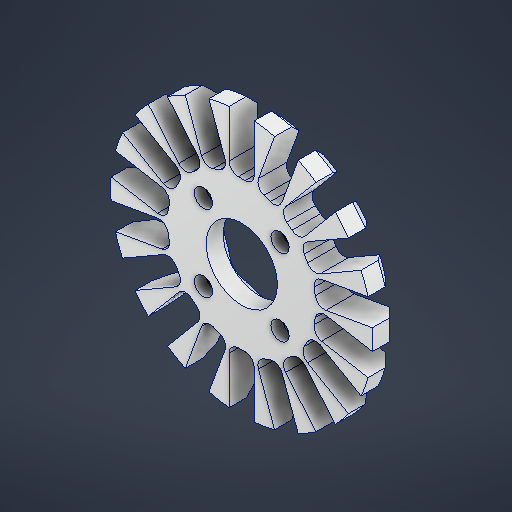
# Autodesk Inventor part: Raddeckel
Saved by Autodesk Inventor 2025.2 (Build 292293000, 293)
## iProperties
Created: 2025-03-24
Part Number: Raddeckel
Material: Generisch
Document SubType Name: Modeling
Designer: Faabs
Density: 1 g/cm^3
Appearance: Aluminium - flach
Author: Faabs
Autodesk Inventor part; units mm, degrees
ref_plane "YZ Plane" through (0, 0, 0) normal (1, 0, 0) x (0, 1, 0)
ref_plane "XZ Plane" through (0, 0, 0) normal (0, 1, 0) x (-1, 0, 0)
ref_plane "XY Plane" through (0, 0, 0) normal (0, 0, 1) x (1, 0, 0)
sketch "Skizze1" plane through (0, 0, 0) normal (0, 0, 1) x (1, 0, 0)
  line L0 (0, 0) -> (0, 5)
  line L1 (0, 0) -> (23, 0)
  line L2 (23, 0) -> (23, 3)
  line L3 (6.25, 0) -> (6.25, 5)
  line L4 (6.25, 5) -> (21, 5)
  line L5 (21, 5) -> (23, 3)
  dimension "d0" = 5
  dimension "d1" = 23
  dimension "d2" = 5
  dimension "d3" = 12.5
  dimension "d4" = 3
  dimension "d5" = 46
  dimension "d6" = 45
  constraints: 12 end point, 3 vertical, 2 horizontal, 2 point on line
  measures "d0" distance of L0.start L0.end
  measures "d1" distance of L0.start L1.end
  measures "d2" distance of L3.start L3.end
  measures "d3" diameter of L3 L0
  measures "d4" distance of L2.start L2.end
  measures "d5" diameter of L2 L0
  measures "d6" angle of L2 L5
revolve "Radkörper" add sketch "Skizze1" angle 360 about axis through (0, 0, 0) along (0, 1, 0)
sketch "Skizze2" plane through (0, 0, 0) normal (0, -1, 0) x (1, 0, 0)
  circle A0 centre (0, 0) radius 23
  circle A1 centre (0, 0) radius 13 construction
  line L0 (0, 0) -> (0, 23) construction
  line L1 (0, 23) -> (2.2, 23)
  line L2 (2.2, 23) -> (2.2, 14.6)
  line L3 (0.6, 13) -> (0, 13)
  line L4 (0, 13) -> (0, 23) construction
  line L5 (0, 23) -> (-2.2, 23)
  line L6 (-2.2, 23) -> (-2.2, 14.6)
  line L7 (-0.6, 13) -> (0, 13)
  line L8 (0, 13) -> (0, 23) construction
  arc A2 (-2.2, 14.6) -> (-0.6, 13) centre (-0.6, 14.6) ccw
  arc A3 (0.6, 13) -> (2.2, 14.6) centre (0.6, 14.6) ccw
  point P0 (2.2, 13)
  point P1 (-2.2, 13)
  point P2 (2.2, 22.8945)
  point P3 (-2.2, 22.8945)
  point P4 (0, 13)
  dimension "d8" = 46
  dimension "d9" = 26
  dimension "d10" = 2.2
  dimension "d12" = 4.4
  dimension "d15" = 1.6
  dimension "d46" = 8.4
  dimension "d47" = 8.4
  constraints: 18 end point, 4 parallel, 4 point on circle, 4 point on line, 4 tangent, 3 centre point, 2 coincident, 2 horizontal, 2 perpendicular, 1 equal radius, 1 vertical, 3 other
  measures "d9" diameter of A1
  measures "d10" distance of point (2.2, 13) L3.end
  measures "d12" distance between parallel lines of L6 L2
  measures "d15" radius of A2
  measures "d46" distance from line of L1 A3.centre
  measures "d47" distance from line of A2.centre L5
extrude "Querrolle" cut sketch "Skizze2" against normal up to surface (5 mm away) contours L2 A3 L3 L7 A2 L6 A0 picked at (0, 17.4)
pattern_circular "Runde Anordnung1" count 18 over 360 about axis through (0, -10, 0) along (0, 1, 0) of "Querrolle"
sketch "Skizze3" plane through (-2.2, 5, 20.8844) normal (0, 1, 0) x (1, 0, 0)
  circle A0 centre (2.2, 20.8844) radius 9.5 construction
  line L0 (2.2, 20.8844) -> (2.2, 11.3844) construction
  line L1 (2.2, 20.8844) -> (8.9175, 14.1669) construction
  point P0 (8.9175, 27.602)
  point P1 (-4.5175, 27.602)
  point P2 (-4.5175, 14.1669)
  dimension "d21" = 19
  dimension "d22" = 45
  dimension "d25" = 360
  constraints: 4 end point, 2 coincident, 2 point on circle, 1 centre point, 1 vertical, 5 other
  measures "d21" diameter of A0
  measures "d22" angle of L1 L0
hole "Bohrung1" at (6.7175, 5, 6.7175) at (6.7175, 5, -6.7175) at (-6.7175, 5, -6.7175) at (-6.7175, 5, 6.7175) direction (0, -1, 0) diameter 3.2 depth 5 tip angle 118 counterbore diameter 5.6 counterbore depth 3
chamfer "Fasen5" distance 2 angle 45 1 edges at (-6.25, 5, 0)
chamfer "Fasen6" distance 0.25 angle 45 6 edges at (-4.9297, 5, 8.8724) (-9.5055, 5, 6.9771) (4.9297, 5, 8.8724) (9.5055, 5, 6.9771) (-8.6974, 5, -8.6974) (8.6974, 5, -8.6974)
sketch "Skizze5" plane through (-2.2, 5, 20.8844) normal (0, 1, 0) x (1, 0, 0)
  circle A0 centre (2.2, 20.8844) radius 6.25
  constraints: 1 centre point, 1 coincident
extrude "Extrusion3" [suppressed]
sketch "Skizze6" plane through (-2.2, 5, 20.8844) normal (0, 1, 0) x (1, 0, 0)
  circle A0 centre (3.6842, 23.4177) radius 1
  circle A1 centre (4.7424, 19.8077) radius 1
  circle A2 centre (1.6362, 17.6858) radius 1
  circle A3 centre (-1.3418, 19.9843) radius 1
  circle A4 centre (-0.076, 23.5268) radius 1
  circle A5 centre (1.729, 20.8844) radius 1.6
  line L0 (1.729, 20.8844) -> (2.2, 20.8844)
  circle A6 centre (1.729, 20.8844) radius 1.6
  spline S0 degree 5 poles (4.0455, 16.9262) (4.0402, 16.9231) (4.0297, 16.9169) (4.014, 16.9073) (3.9934, 16.894) (3.9682, 16.8764) (3.9436, 16.8581) (3.9196, 16.8389) (3.8963, 16.8192) (3.8739, 16.799) (3.8525, 16.7785) (3.8322, 16.758) (3.813, 16.7376) (3.7948, 16.7171) (3.7774, 16.6963) (3.7607, 16.675) (3.7442, 16.6528) (3.7279, 16.6295) (3.7116, 16.6049) (3.6956, 16.579) (3.6799, 16.5519) (3.6648, 16.5239) (3.6505, 16.4953) (3.6371, 16.4663) (3.6248, 16.4374) (3.6136, 16.4089) (3.6035, 16.3809) (3.5944, 16.3536) (3.5861, 16.3267) (3.5786, 16.2999) (3.5716, 16.2728) (3.565, 16.2453) (3.5586, 16.2172) (3.5524, 16.1887) (3.5463, 16.1602) (3.5403, 16.132) (3.534, 16.1044) (3.527, 16.0771) (3.5186, 16.0497) (3.5081, 16.0214) (3.495, 15.9919) (3.4788, 15.9607) (3.4596, 15.928) (3.4382, 15.8946) (3.4152, 15.8615) (3.3915, 15.8297) (3.368, 15.8004) (3.3452, 15.774) (3.3233, 15.7507) (3.302, 15.73) (3.2808, 15.7111) (3.2589, 15.693) (3.2359, 15.675) (3.2114, 15.6567) (3.1855, 15.6381) (3.1584, 15.6194) (3.1303, 15.601) (3.1015, 15.5835) (3.0723, 15.5669) (3.0427, 15.5515) (3.0127, 15.5372) (2.9823, 15.5238) (2.9513, 15.5112) (2.9198, 15.4994) (2.8876, 15.4883) (2.855, 15.4779) (2.822, 15.4683) (2.7887, 15.4596) (2.7552, 15.4518) (2.7215, 15.445) (2.6876, 15.4393) (2.6536, 15.4346) (2.6196, 15.4309) (2.5854, 15.4283) (2.5512, 15.4266) (2.517, 15.4258) (2.483, 15.426) (2.4493, 15.427) (2.4158, 15.4288) (2.3827, 15.4316) (2.3499, 15.4352) (2.3173, 15.4399) (2.285, 15.4457) (2.2528, 15.4525) (2.221, 15.4604) (2.1895, 15.4692) (2.1589, 15.4787) (2.1292, 15.4885) (2.1009, 15.4987) (2.0737, 15.5091) (2.0476, 15.52) (2.022, 15.5318) (1.9962, 15.545) (1.9698, 15.56) (1.9426, 15.5769) (1.9149, 15.5955) (1.8875, 15.6151) (1.8612, 15.635) (1.8369, 15.6545) (1.815, 15.6734) (1.7956, 15.6918) (1.778, 15.7104) (1.7615, 15.7301) (1.7452, 15.7516) (1.7285, 15.7754) (1.7111, 15.8014) (1.693, 15.829) (1.6745, 15.8575) (1.6557, 15.8862) (1.6368, 15.9144) (1.6177, 15.9418) (1.598, 15.9686) (1.5775, 15.9948) (1.5559, 16.0206) (1.5331, 16.0461) (1.5093, 16.0711) (1.4849, 16.0953) (1.4605, 16.1182) (1.4366, 16.1394) (1.4135, 16.1587) (1.3913, 16.1761) (1.3698, 16.1919) (1.3485, 16.2067) (1.3267, 16.2209) (1.3039, 16.2351) (1.2796, 16.2494) (1.2537, 16.2637) (1.2259, 16.2778) (1.1964, 16.2915) (1.1657, 16.3044) (1.1343, 16.3164) (1.1031, 16.3272) (1.0728, 16.3367) (1.0443, 16.3449) (1.0183, 16.3517) (0.9953, 16.3571) (0.9793, 16.3603) (0.9687, 16.362) (0.9623, 16.3629) (0.9593, 16.3632) knots 0 0 0 0 0 0 0.007407 0.014815 0.022222 0.02963 0.037037 0.044444 0.051852 0.059259 0.066667 0.074074 0.081481 0.088889 0.096296 0.103704 0.111111 0.118519 0.125926 0.133333 0.140741 0.148148 0.155556 0.162963 0.17037 0.177778 0.185185 0.192593 0.2 0.207407 0.214815 0.222222 0.22963 0.237037 0.244444 0.251852 0.259259 0.266667 0.274074 0.281481 0.288889 0.296296 0.303704 0.311111 0.318519 0.325926 0.333333 0.340741 0.348148 0.355556 0.362963 0.37037 0.377778 0.385185 0.392593 0.4 0.407407 0.414815 0.422222 0.42963 0.437037 0.444444 0.451852 0.459259 0.466667 0.474074 0.481481 0.488889 0.496296 0.503704 0.511111 0.518519 0.525926 0.533333 0.540741 0.548148 0.555556 0.562963 0.57037 0.577778 0.585185 0.592593 0.6 0.607407 0.614815 0.622222 0.62963 0.637037 0.644444 0.651852 0.659259 0.666667 0.674074 0.681481 0.688889 0.696296 0.703704 0.711111 0.718519 0.725926 0.733333 0.740741 0.748148 0.755556 0.762963 0.77037 0.777778 0.785185 0.792593 0.8 0.807407 0.814815 0.822222 0.82963 0.837037 0.844444 0.851852 0.859259 0.866667 0.874074 0.881481 0.888889 0.896296 0.903704 0.911111 0.918519 0.925926 0.933333 0.940741 0.948148 0.955556 0.962963 0.97037 0.977778 0.985185 0.992593 1 1 1 1 1 1
  spline S1 degree 5 poles (0.9593, 16.3632) (0.9532, 16.3643) (0.9411, 16.3663) (0.9229, 16.369) (0.8986, 16.3721) (0.868, 16.3748) (0.8374, 16.3766) (0.8067, 16.3773) (0.7762, 16.3771) (0.746, 16.3761) (0.7165, 16.3742) (0.6877, 16.3715) (0.6598, 16.3682) (0.6327, 16.3642) (0.6061, 16.3594) (0.5796, 16.3539) (0.5527, 16.3475) (0.5252, 16.3401) (0.4969, 16.3317) (0.468, 16.3222) (0.4386, 16.3116) (0.409, 16.2998) (0.3796, 16.2871) (0.3508, 16.2735) (0.3228, 16.2592) (0.2959, 16.2445) (0.2701, 16.2296) (0.2456, 16.2145) (0.222, 16.1992) (0.199, 16.1836) (0.1762, 16.1674) (0.1534, 16.1505) (0.1305, 16.1331) (0.1074, 16.1152) (0.0845, 16.0973) (0.0617, 16.0796) (0.0391, 16.0624) (0.0162, 16.046) (-0.0078, 16.0304) (-0.034, 16.0156) (-0.0631, 16.0014) (-0.0956, 15.9879) (-0.1312, 15.9751) (-0.1691, 15.9633) (-0.208, 15.9528) (-0.2466, 15.9437) (-0.2835, 15.9363) (-0.3178, 15.9307) (-0.3496, 15.927) (-0.3792, 15.9248) (-0.4076, 15.924) (-0.436, 15.9242) (-0.4652, 15.9252) (-0.4957, 15.9269) (-0.5276, 15.9293) (-0.5604, 15.9324) (-0.5937, 15.9364) (-0.627, 15.9414) (-0.66, 15.9475) (-0.6926, 15.9547) (-0.7248, 15.963) (-0.7567, 15.9723) (-0.7885, 15.9826) (-0.8203, 15.9939) (-0.852, 16.006) (-0.8837, 16.019) (-0.9151, 16.0328) (-0.9463, 16.0476) (-0.977, 16.0632) (-1.0071, 16.0797) (-1.0367, 16.097) (-1.0658, 16.1153) (-1.0942, 16.1344) (-1.1221, 16.1543) (-1.1494, 16.175) (-1.1761, 16.1964) (-1.202, 16.2183) (-1.2273, 16.2408) (-1.2517, 16.2637) (-1.2753, 16.2871) (-1.2981, 16.311) (-1.32, 16.3355) (-1.3411, 16.3607) (-1.3613, 16.3866) (-1.3806, 16.4132) (-1.3991, 16.4401) (-1.4165, 16.4671) (-1.4328, 16.4937) (-1.448, 16.5197) (-1.4621, 16.5451) (-1.4751, 16.5702) (-1.4872, 16.5957) (-1.4985, 16.6224) (-1.5091, 16.6509) (-1.519, 16.6814) (-1.5283, 16.7134) (-1.5367, 16.746) (-1.544, 16.7781) (-1.5501, 16.8088) (-1.5547, 16.8373) (-1.5578, 16.8639) (-1.5592, 16.8894) (-1.5592, 16.9151) (-1.5579, 16.942) (-1.5554, 16.971) (-1.552, 17.0021) (-1.5481, 17.0349) (-1.544, 17.0686) (-1.54, 17.1026) (-1.5363, 17.1364) (-1.5333, 17.1697) (-1.5312, 17.2029) (-1.5301, 17.2361) (-1.53, 17.2698) (-1.5311, 17.304) (-1.5333, 17.3384) (-1.5364, 17.3726) (-1.5404, 17.4058) (-1.545, 17.4375) (-1.5503, 17.4671) (-1.5561, 17.4947) (-1.5624, 17.5206) (-1.5693, 17.5457) (-1.5768, 17.5706) (-1.5852, 17.5961) (-1.5946, 17.6226) (-1.6053, 17.6503) (-1.6175, 17.679) (-1.6313, 17.7084) (-1.6465, 17.738) (-1.6628, 17.7674) (-1.6798, 17.7957) (-1.6969, 17.8225) (-1.7134, 17.8471) (-1.729, 17.869) (-1.7432, 17.888) (-1.7534, 17.9006) (-1.7604, 17.9088) (-1.7647, 17.9135) (-1.7668, 17.9158) knots 0 0 0 0 0 0 0.007407 0.014815 0.022222 0.02963 0.037037 0.044444 0.051852 0.059259 0.066667 0.074074 0.081481 0.088889 0.096296 0.103704 0.111111 0.118519 0.125926 0.133333 0.140741 0.148148 0.155556 0.162963 0.17037 0.177778 0.185185 0.192593 0.2 0.207407 0.214815 0.222222 0.22963 0.237037 0.244444 0.251852 0.259259 0.266667 0.274074 0.281481 0.288889 0.296296 0.303704 0.311111 0.318519 0.325926 0.333333 0.340741 0.348148 0.355556 0.362963 0.37037 0.377778 0.385185 0.392593 0.4 0.407407 0.414815 0.422222 0.42963 0.437037 0.444444 0.451852 0.459259 0.466667 0.474074 0.481481 0.488889 0.496296 0.503704 0.511111 0.518519 0.525926 0.533333 0.540741 0.548148 0.555556 0.562963 0.57037 0.577778 0.585185 0.592593 0.6 0.607407 0.614815 0.622222 0.62963 0.637037 0.644444 0.651852 0.659259 0.666667 0.674074 0.681481 0.688889 0.696296 0.703704 0.711111 0.718519 0.725926 0.733333 0.740741 0.748148 0.755556 0.762963 0.77037 0.777778 0.785185 0.792593 0.8 0.807407 0.814815 0.822222 0.82963 0.837037 0.844444 0.851852 0.859259 0.866667 0.874074 0.881481 0.888889 0.896296 0.903704 0.911111 0.918519 0.925926 0.933333 0.940741 0.948148 0.955556 0.962963 0.97037 0.977778 0.985185 0.992593 1 1 1 1 1 1
  spline S2 degree 5 poles (-1.7668, 17.9158) (-1.7708, 17.9205) (-1.7787, 17.9298) (-1.7909, 17.9436) (-1.8076, 17.9615) (-1.8293, 17.9833) (-1.8516, 18.0043) (-1.8747, 18.0246) (-1.8982, 18.0441) (-1.9219, 18.0627) (-1.9458, 18.0802) (-1.9695, 18.0967) (-1.993, 18.112) (-2.0164, 18.1264) (-2.0398, 18.1399) (-2.0637, 18.1527) (-2.0884, 18.165) (-2.1142, 18.1771) (-2.1413, 18.1888) (-2.1696, 18.2001) (-2.1989, 18.2109) (-2.2291, 18.2209) (-2.2598, 18.23) (-2.2906, 18.2381) (-2.3213, 18.2452) (-2.3513, 18.2513) (-2.3806, 18.2564) (-2.4091, 18.2606) (-2.4371, 18.2641) (-2.4647, 18.2668) (-2.4926, 18.269) (-2.5208, 18.2708) (-2.5497, 18.2722) (-2.5788, 18.2734) (-2.6079, 18.2744) (-2.6367, 18.2754) (-2.665, 18.2768) (-2.6931, 18.2789) (-2.7216, 18.2825) (-2.7512, 18.2879) (-2.7826, 18.2957) (-2.8161, 18.3063) (-2.8516, 18.3194) (-2.8883, 18.3347) (-2.9249, 18.3517) (-2.9602, 18.3695) (-2.9932, 18.3875) (-3.0232, 18.4054) (-3.0499, 18.4229) (-3.0739, 18.4402) (-3.0963, 18.4579) (-3.1179, 18.4763) (-3.1396, 18.4958) (-3.1619, 18.5168) (-3.1848, 18.539) (-3.2079, 18.5625) (-3.2308, 18.587) (-3.2531, 18.6123) (-3.2745, 18.6381) (-3.2948, 18.6646) (-3.3141, 18.6917) (-3.3326, 18.7193) (-3.3503, 18.7476) (-3.3675, 18.7767) (-3.384, 18.8064) (-3.3999, 18.8367) (-3.4151, 18.8675) (-3.4295, 18.8988) (-3.4429, 18.9305) (-3.4555, 18.9625) (-3.467, 18.9949) (-3.4775, 19.0275) (-3.487, 19.0604) (-3.4956, 19.0936) (-3.5032, 19.127) (-3.5099, 19.1605) (-3.5156, 19.194) (-3.5205, 19.2274) (-3.5245, 19.2607) (-3.5275, 19.2938) (-3.5296, 19.3267) (-3.5307, 19.3596) (-3.5306, 19.3925) (-3.5294, 19.4253) (-3.5272, 19.4581) (-3.524, 19.4906) (-3.52, 19.5224) (-3.5154, 19.5533) (-3.5104, 19.583) (-3.5049, 19.6115) (-3.4987, 19.6391) (-3.4915, 19.6664) (-3.483, 19.6941) (-3.4728, 19.7228) (-3.4608, 19.7525) (-3.4473, 19.783) (-3.4328, 19.8134) (-3.4178, 19.8427) (-3.4027, 19.8701) (-3.3879, 19.8949) (-3.3732, 19.9172) (-3.3579, 19.9377) (-3.3414, 19.9574) (-3.323, 19.9771) (-3.3025, 19.9977) (-3.2799, 20.0194) (-3.2559, 20.042) (-3.231, 20.0652) (-3.2061, 20.0886) (-3.1816, 20.1122) (-3.1579, 20.1358) (-3.1349, 20.1598) (-3.1127, 20.1846) (-3.091, 20.2103) (-3.0699, 20.2372) (-3.0494, 20.265) (-3.0298, 20.2932) (-3.0115, 20.3212) (-2.9947, 20.3484) (-2.9797, 20.3745) (-2.9665, 20.3994) (-2.9546, 20.4233) (-2.9438, 20.4469) (-2.9335, 20.4708) (-2.9235, 20.4957) (-2.9137, 20.5221) (-2.9041, 20.5502) (-2.895, 20.58) (-2.8866, 20.6114) (-2.8792, 20.6439) (-2.8729, 20.6769) (-2.8677, 20.7095) (-2.8636, 20.741) (-2.8604, 20.7704) (-2.8583, 20.7972) (-2.857, 20.8209) (-2.8566, 20.8372) (-2.8568, 20.8479) (-2.857, 20.8543) (-2.8572, 20.8574) knots 0 0 0 0 0 0 0.007407 0.014815 0.022222 0.02963 0.037037 0.044444 0.051852 0.059259 0.066667 0.074074 0.081481 0.088889 0.096296 0.103704 0.111111 0.118519 0.125926 0.133333 0.140741 0.148148 0.155556 0.162963 0.17037 0.177778 0.185185 0.192593 0.2 0.207407 0.214815 0.222222 0.22963 0.237037 0.244444 0.251852 0.259259 0.266667 0.274074 0.281481 0.288889 0.296296 0.303704 0.311111 0.318519 0.325926 0.333333 0.340741 0.348148 0.355556 0.362963 0.37037 0.377778 0.385185 0.392593 0.4 0.407407 0.414815 0.422222 0.42963 0.437037 0.444444 0.451852 0.459259 0.466667 0.474074 0.481481 0.488889 0.496296 0.503704 0.511111 0.518519 0.525926 0.533333 0.540741 0.548148 0.555556 0.562963 0.57037 0.577778 0.585185 0.592593 0.6 0.607407 0.614815 0.622222 0.62963 0.637037 0.644444 0.651852 0.659259 0.666667 0.674074 0.681481 0.688889 0.696296 0.703704 0.711111 0.718519 0.725926 0.733333 0.740741 0.748148 0.755556 0.762963 0.77037 0.777778 0.785185 0.792593 0.8 0.807407 0.814815 0.822222 0.82963 0.837037 0.844444 0.851852 0.859259 0.866667 0.874074 0.881481 0.888889 0.896296 0.903704 0.911111 0.918519 0.925926 0.933333 0.940741 0.948148 0.955556 0.962963 0.97037 0.977778 0.985185 0.992593 1 1 1 1 1 1
  spline S3 degree 5 poles (-2.8572, 20.8574) (-2.8572, 20.8635) (-2.8573, 20.8758) (-2.8578, 20.8942) (-2.859, 20.9187) (-2.8616, 20.9493) (-2.8652, 20.9798) (-2.8698, 21.0101) (-2.8753, 21.0401) (-2.8816, 21.0696) (-2.8886, 21.0984) (-2.8962, 21.1262) (-2.9043, 21.1531) (-2.913, 21.1791) (-2.9223, 21.2045) (-2.9323, 21.2297) (-2.9433, 21.2551) (-2.9553, 21.2809) (-2.9685, 21.3072) (-2.9829, 21.3341) (-2.9985, 21.3612) (-3.0152, 21.3883) (-3.0328, 21.415) (-3.0512, 21.441) (-3.0701, 21.4661) (-3.0893, 21.4901) (-3.1084, 21.5128) (-3.1276, 21.5344) (-3.1467, 21.555) (-3.1662, 21.5749) (-3.1861, 21.5945) (-3.2066, 21.614) (-3.2278, 21.6336) (-3.2493, 21.6532) (-3.271, 21.6727) (-3.2924, 21.692) (-3.3132, 21.7113) (-3.3333, 21.731) (-3.3529, 21.752) (-3.372, 21.7752) (-3.3911, 21.8014) (-3.41, 21.831) (-3.4287, 21.8639) (-3.4469, 21.8992) (-3.4641, 21.9357) (-3.4798, 21.972) (-3.4934, 22.0071) (-3.5049, 22.04) (-3.5141, 22.0706) (-3.5214, 22.0994) (-3.5271, 22.1272) (-3.5319, 22.1552) (-3.5359, 22.1841) (-3.5396, 22.2145) (-3.5428, 22.2463) (-3.5454, 22.2791) (-3.5472, 22.3126) (-3.548, 22.3463) (-3.5478, 22.3798) (-3.5463, 22.4132) (-3.5438, 22.4463) (-3.5401, 22.4794) (-3.5355, 22.5125) (-3.53, 22.5457) (-3.5235, 22.5791) (-3.5162, 22.6126) (-3.5081, 22.6459) (-3.4989, 22.6792) (-3.4889, 22.7121) (-3.4779, 22.7447) (-3.466, 22.7768) (-3.453, 22.8086) (-3.4392, 22.84) (-3.4244, 22.8709) (-3.4087, 22.9013) (-3.3923, 22.9313) (-3.3752, 22.9607) (-3.3575, 22.9894) (-3.3391, 23.0175) (-3.3202, 23.0448) (-3.3006, 23.0714) (-3.2803, 23.0972) (-3.2591, 23.1223) (-3.2371, 23.1467) (-3.2143, 23.1704) (-3.191, 23.1932) (-3.1675, 23.2151) (-3.1441, 23.2358) (-3.1211, 23.2553) (-3.0986, 23.2736) (-3.0761, 23.2907) (-3.053, 23.3071) (-3.0287, 23.3228) (-3.0025, 23.3382) (-2.9742, 23.3533) (-2.9443, 23.3679) (-2.9136, 23.3819) (-2.8833, 23.3947) (-2.8542, 23.406) (-2.8269, 23.4155) (-2.8012, 23.4231) (-2.7763, 23.429) (-2.7511, 23.4334) (-2.7243, 23.4368) (-2.6953, 23.4394) (-2.6641, 23.4415) (-2.6311, 23.4433) (-2.5972, 23.4451) (-2.563, 23.447) (-2.5291, 23.4493) (-2.4958, 23.4522) (-2.4628, 23.4558) (-2.4298, 23.4605) (-2.3967, 23.4663) (-2.3632, 23.4733) (-2.3297, 23.4814) (-2.2965, 23.4904) (-2.2645, 23.5001) (-2.2341, 23.5102) (-2.2059, 23.5205) (-2.1797, 23.531) (-2.1553, 23.5418) (-2.1318, 23.5529) (-2.1086, 23.5646) (-2.0849, 23.5773) (-2.0604, 23.5911) (-2.035, 23.6065) (-2.0089, 23.6235) (-1.9823, 23.6421) (-1.9557, 23.6623) (-1.9297, 23.6835) (-1.9047, 23.7052) (-1.8813, 23.7266) (-1.86, 23.7471) (-1.8411, 23.7662) (-1.8249, 23.7835) (-1.8142, 23.7958) (-1.8074, 23.8041) (-1.8035, 23.8092) (-1.8016, 23.8117) knots 0 0 0 0 0 0 0.007407 0.014815 0.022222 0.02963 0.037037 0.044444 0.051852 0.059259 0.066667 0.074074 0.081481 0.088889 0.096296 0.103704 0.111111 0.118519 0.125926 0.133333 0.140741 0.148148 0.155556 0.162963 0.17037 0.177778 0.185185 0.192593 0.2 0.207407 0.214815 0.222222 0.22963 0.237037 0.244444 0.251852 0.259259 0.266667 0.274074 0.281481 0.288889 0.296296 0.303704 0.311111 0.318519 0.325926 0.333333 0.340741 0.348148 0.355556 0.362963 0.37037 0.377778 0.385185 0.392593 0.4 0.407407 0.414815 0.422222 0.42963 0.437037 0.444444 0.451852 0.459259 0.466667 0.474074 0.481481 0.488889 0.496296 0.503704 0.511111 0.518519 0.525926 0.533333 0.540741 0.548148 0.555556 0.562963 0.57037 0.577778 0.585185 0.592593 0.6 0.607407 0.614815 0.622222 0.62963 0.637037 0.644444 0.651852 0.659259 0.666667 0.674074 0.681481 0.688889 0.696296 0.703704 0.711111 0.718519 0.725926 0.733333 0.740741 0.748148 0.755556 0.762963 0.77037 0.777778 0.785185 0.792593 0.8 0.807407 0.814815 0.822222 0.82963 0.837037 0.844444 0.851852 0.859259 0.866667 0.874074 0.881481 0.888889 0.896296 0.903704 0.911111 0.918519 0.925926 0.933333 0.940741 0.948148 0.955556 0.962963 0.97037 0.977778 0.985185 0.992593 1 1 1 1 1 1
  spline S4 degree 5 poles (-1.8016, 23.8117) (-1.7977, 23.8164) (-1.7899, 23.8258) (-1.7784, 23.8402) (-1.7636, 23.8598) (-1.746, 23.8849) (-1.7291, 23.9106) (-1.7131, 23.9367) (-1.698, 23.9633) (-1.6839, 23.9899) (-1.6708, 24.0164) (-1.6587, 24.0427) (-1.6476, 24.0685) (-1.6375, 24.094) (-1.6283, 24.1194) (-1.6199, 24.1452) (-1.612, 24.1717) (-1.6046, 24.1992) (-1.5978, 24.2278) (-1.5915, 24.2577) (-1.586, 24.2884) (-1.5814, 24.3199) (-1.5778, 24.3517) (-1.5751, 24.3835) (-1.5735, 24.4149) (-1.5727, 24.4455) (-1.5728, 24.4753) (-1.5736, 24.5041) (-1.575, 24.5322) (-1.5771, 24.5599) (-1.5797, 24.5877) (-1.5829, 24.6159) (-1.5865, 24.6445) (-1.5905, 24.6734) (-1.5945, 24.7022) (-1.5985, 24.7308) (-1.6021, 24.7589) (-1.6048, 24.7869) (-1.6063, 24.8156) (-1.6061, 24.8457) (-1.6038, 24.878) (-1.5993, 24.9128) (-1.5925, 24.9501) (-1.5837, 24.9888) (-1.5734, 25.0278) (-1.5621, 25.0657) (-1.55, 25.1014) (-1.5376, 25.1339) (-1.525, 25.1633) (-1.5121, 25.19) (-1.4986, 25.2151) (-1.4842, 25.2395) (-1.4687, 25.2643) (-1.452, 25.2899) (-1.4341, 25.3163) (-1.4149, 25.3431) (-1.3948, 25.37) (-1.3738, 25.3963) (-1.352, 25.4218) (-1.3295, 25.4464) (-1.3062, 25.4702) (-1.2822, 25.4932) (-1.2574, 25.5156) (-1.2318, 25.5375) (-1.2054, 25.5589) (-1.1783, 25.5798) (-1.1506, 25.6001) (-1.1222, 25.6197) (-1.0934, 25.6385) (-1.064, 25.6564) (-1.0342, 25.6734) (-1.0038, 25.6894) (-0.9731, 25.7045) (-0.9419, 25.7187) (-0.9103, 25.732) (-0.8785, 25.7444) (-0.8465, 25.7559) (-0.8144, 25.7665) (-0.7823, 25.7762) (-0.7503, 25.7849) (-0.7182, 25.7927) (-0.686, 25.7994) (-0.6536, 25.8051) (-0.6211, 25.8096) (-0.5884, 25.8131) (-0.5559, 25.8156) (-0.5238, 25.8172) (-0.4926, 25.8181) (-0.4625, 25.8182) (-0.4335, 25.8177) (-0.4052, 25.8165) (-0.377, 25.8141) (-0.3483, 25.8105) (-0.3183, 25.8055) (-0.287, 25.7988) (-0.2546, 25.7909) (-0.2222, 25.7818) (-0.1907, 25.7721) (-0.1611, 25.7621) (-0.1341, 25.7518) (-0.1095, 25.7412) (-0.0867, 25.7297) (-0.0645, 25.7168) (-0.0418, 25.7022) (-0.0179, 25.6855) (0.0073, 25.6671) (0.0337, 25.6473) (0.0609, 25.6269) (0.0883, 25.6064) (0.1157, 25.5863) (0.1431, 25.5671) (0.1708, 25.5487) (0.199, 25.5311) (0.2281, 25.5142) (0.2582, 25.498) (0.2892, 25.4827) (0.3203, 25.4683) (0.3511, 25.4551) (0.3809, 25.4433) (0.4092, 25.4331) (0.4359, 25.4243) (0.4616, 25.4168) (0.4867, 25.4103) (0.512, 25.4043) (0.5383, 25.3988) (0.566, 25.3937) (0.5953, 25.3891) (0.6262, 25.3854) (0.6586, 25.3826) (0.6919, 25.3809) (0.7255, 25.3804) (0.7585, 25.381) (0.7902, 25.3823) (0.8198, 25.3844) (0.8465, 25.3869) (0.87, 25.3897) (0.8861, 25.3922) (0.8967, 25.3942) (0.903, 25.3956) (0.906, 25.3963) knots 0 0 0 0 0 0 0.007407 0.014815 0.022222 0.02963 0.037037 0.044444 0.051852 0.059259 0.066667 0.074074 0.081481 0.088889 0.096296 0.103704 0.111111 0.118519 0.125926 0.133333 0.140741 0.148148 0.155556 0.162963 0.17037 0.177778 0.185185 0.192593 0.2 0.207407 0.214815 0.222222 0.22963 0.237037 0.244444 0.251852 0.259259 0.266667 0.274074 0.281481 0.288889 0.296296 0.303704 0.311111 0.318519 0.325926 0.333333 0.340741 0.348148 0.355556 0.362963 0.37037 0.377778 0.385185 0.392593 0.4 0.407407 0.414815 0.422222 0.42963 0.437037 0.444444 0.451852 0.459259 0.466667 0.474074 0.481481 0.488889 0.496296 0.503704 0.511111 0.518519 0.525926 0.533333 0.540741 0.548148 0.555556 0.562963 0.57037 0.577778 0.585185 0.592593 0.6 0.607407 0.614815 0.622222 0.62963 0.637037 0.644444 0.651852 0.659259 0.666667 0.674074 0.681481 0.688889 0.696296 0.703704 0.711111 0.718519 0.725926 0.733333 0.740741 0.748148 0.755556 0.762963 0.77037 0.777778 0.785185 0.792593 0.8 0.807407 0.814815 0.822222 0.82963 0.837037 0.844444 0.851852 0.859259 0.866667 0.874074 0.881481 0.888889 0.896296 0.903704 0.911111 0.918519 0.925926 0.933333 0.940741 0.948148 0.955556 0.962963 0.97037 0.977778 0.985185 0.992593 1 1 1 1 1 1
  spline S5 degree 5 poles (0.906, 25.3963) (0.912, 25.3973) (0.9241, 25.3996) (0.9421, 25.4032) (0.966, 25.4087) (0.9957, 25.4166) (1.0251, 25.4254) (1.0542, 25.4352) (1.0828, 25.4458) (1.1107, 25.4571) (1.1379, 25.469) (1.164, 25.4813) (1.189, 25.494) (1.2131, 25.507) (1.2365, 25.5206) (1.2596, 25.5349) (1.2826, 25.5501) (1.306, 25.5665) (1.3297, 25.584) (1.3536, 25.6029) (1.3776, 25.6229) (1.4014, 25.644) (1.4246, 25.6661) (1.447, 25.6887) (1.4685, 25.7117) (1.4888, 25.7347) (1.5078, 25.7575) (1.5258, 25.7801) (1.5427, 25.8026) (1.559, 25.8251) (1.5748, 25.8481) (1.5904, 25.8717) (1.6061, 25.896) (1.6216, 25.9206) (1.6371, 25.9454) (1.6524, 25.9698) (1.6677, 25.9936) (1.6836, 26.0169) (1.7009, 26.0397) (1.7204, 26.0627) (1.7429, 26.0859) (1.7688, 26.1097) (1.7979, 26.1339) (1.8295, 26.158) (1.8625, 26.1812) (1.8956, 26.2029) (1.9277, 26.2225) (1.9581, 26.2395) (1.9867, 26.2539) (2.0137, 26.266) (2.0402, 26.2765) (2.0669, 26.286) (2.0947, 26.2951) (2.124, 26.3039) (2.1547, 26.3126) (2.1866, 26.3209) (2.2193, 26.3285) (2.2523, 26.3352) (2.2854, 26.3407) (2.3185, 26.3451) (2.3516, 26.3483) (2.3847, 26.3505) (2.4182, 26.3517) (2.4519, 26.352) (2.4858, 26.3515) (2.52, 26.3501) (2.5543, 26.3478) (2.5886, 26.3446) (2.6228, 26.3404) (2.6568, 26.3353) (2.6906, 26.3291) (2.7241, 26.3219) (2.7574, 26.3137) (2.7904, 26.3045) (2.8231, 26.2944) (2.8555, 26.2834) (2.8874, 26.2716) (2.9187, 26.2591) (2.9496, 26.246) (2.9797, 26.2321) (3.0093, 26.2174) (3.0383, 26.2018) (3.0667, 26.1854) (3.0946, 26.1679) (3.1218, 26.1496) (3.1484, 26.1306) (3.174, 26.1112) (3.1984, 26.0918) (3.2216, 26.0726) (3.2435, 26.0536) (3.2644, 26.0344) (3.2844, 26.0145) (3.3042, 25.9933) (3.3238, 25.9701) (3.3436, 25.9449) (3.3632, 25.918) (3.3823, 25.8902) (3.4002, 25.8625) (3.4164, 25.8358) (3.4305, 25.8106) (3.4424, 25.7867) (3.4526, 25.7632) (3.4613, 25.7391) (3.4693, 25.7133) (3.4768, 25.6852) (3.4843, 25.6548) (3.4919, 25.6227) (3.4995, 25.5896) (3.5074, 25.5562) (3.5155, 25.5233) (3.5241, 25.4909) (3.5334, 25.459) (3.5437, 25.4274) (3.5552, 25.3958) (3.5679, 25.364) (3.5817, 25.3324) (3.5963, 25.3013) (3.6114, 25.2715) (3.6267, 25.2433) (3.6418, 25.2173) (3.6566, 25.1934) (3.6714, 25.1711) (3.6865, 25.15) (3.7021, 25.1291) (3.7186, 25.108) (3.7365, 25.0863) (3.7561, 25.064) (3.7773, 25.0412) (3.8003, 25.0182) (3.8248, 24.9956) (3.8502, 24.9736) (3.8759, 24.9528) (3.901, 24.9334) (3.925, 24.916) (3.9471, 24.9007) (3.9669, 24.8878) (3.9809, 24.8793) (3.9902, 24.8741) (3.9959, 24.8711) (3.9987, 24.8697) knots 0 0 0 0 0 0 0.007407 0.014815 0.022222 0.02963 0.037037 0.044444 0.051852 0.059259 0.066667 0.074074 0.081481 0.088889 0.096296 0.103704 0.111111 0.118519 0.125926 0.133333 0.140741 0.148148 0.155556 0.162963 0.17037 0.177778 0.185185 0.192593 0.2 0.207407 0.214815 0.222222 0.22963 0.237037 0.244444 0.251852 0.259259 0.266667 0.274074 0.281481 0.288889 0.296296 0.303704 0.311111 0.318519 0.325926 0.333333 0.340741 0.348148 0.355556 0.362963 0.37037 0.377778 0.385185 0.392593 0.4 0.407407 0.414815 0.422222 0.42963 0.437037 0.444444 0.451852 0.459259 0.466667 0.474074 0.481481 0.488889 0.496296 0.503704 0.511111 0.518519 0.525926 0.533333 0.540741 0.548148 0.555556 0.562963 0.57037 0.577778 0.585185 0.592593 0.6 0.607407 0.614815 0.622222 0.62963 0.637037 0.644444 0.651852 0.659259 0.666667 0.674074 0.681481 0.688889 0.696296 0.703704 0.711111 0.718519 0.725926 0.733333 0.740741 0.748148 0.755556 0.762963 0.77037 0.777778 0.785185 0.792593 0.8 0.807407 0.814815 0.822222 0.82963 0.837037 0.844444 0.851852 0.859259 0.866667 0.874074 0.881481 0.888889 0.896296 0.903704 0.911111 0.918519 0.925926 0.933333 0.940741 0.948148 0.955556 0.962963 0.97037 0.977778 0.985185 0.992593 1 1 1 1 1 1
  spline S6 degree 5 poles (3.9987, 24.8697) (4.004, 24.8667) (4.0147, 24.8606) (4.0308, 24.8518) (4.0527, 24.8407) (4.0804, 24.8276) (4.1087, 24.8155) (4.1372, 24.8043) (4.166, 24.7941) (4.1947, 24.7847) (4.2231, 24.7764) (4.251, 24.7691) (4.2783, 24.7626) (4.3052, 24.7572) (4.3318, 24.7525) (4.3587, 24.7486) (4.3861, 24.7455) (4.4145, 24.743) (4.4439, 24.7412) (4.4744, 24.7403) (4.5056, 24.7402) (4.5374, 24.7411) (4.5694, 24.743) (4.6011, 24.746) (4.6323, 24.7498) (4.6626, 24.7544) (4.6919, 24.7596) (4.7202, 24.7654) (4.7476, 24.7717) (4.7746, 24.7785) (4.8015, 24.786) (4.8286, 24.794) (4.8562, 24.8025) (4.884, 24.8114) (4.9117, 24.8204) (4.9391, 24.8293) (4.9662, 24.8377) (4.9933, 24.8453) (5.0212, 24.8517) (5.0509, 24.8567) (5.0831, 24.8601) (5.1182, 24.8617) (5.1561, 24.8615) (5.1958, 24.8596) (5.2359, 24.8562) (5.2753, 24.8516) (5.3125, 24.8459) (5.3467, 24.8393) (5.3778, 24.832) (5.4063, 24.8239) (5.4334, 24.815) (5.4599, 24.8051) (5.487, 24.7942) (5.5152, 24.7821) (5.5442, 24.769) (5.574, 24.7548) (5.6039, 24.7397) (5.6335, 24.7236) (5.6624, 24.7066) (5.6906, 24.6886) (5.718, 24.6698) (5.7448, 24.6502) (5.7712, 24.6296) (5.7972, 24.6082) (5.8229, 24.5859) (5.8482, 24.5629) (5.873, 24.5391) (5.8972, 24.5146) (5.9207, 24.4895) (5.9435, 24.4637) (5.9653, 24.4372) (5.9864, 24.4101) (6.0066, 24.3824) (6.026, 24.3542) (6.0446, 24.3254) (6.0623, 24.2962) (6.0792, 24.2667) (6.0952, 24.2369) (6.1103, 24.207) (6.1245, 24.177) (6.1377, 24.1468) (6.1499, 24.1162) (6.1611, 24.0853) (6.1713, 24.0541) (6.1804, 24.0225) (6.1885, 23.9909) (6.1956, 23.9596) (6.2019, 23.929) (6.2073, 23.8994) (6.2118, 23.8707) (6.2155, 23.8426) (6.2181, 23.8145) (6.2195, 23.7855) (6.2197, 23.7552) (6.2187, 23.7231) (6.2164, 23.6899) (6.2132, 23.6564) (6.2091, 23.6237) (6.2043, 23.5928) (6.1989, 23.5644) (6.1927, 23.5384) (6.1853, 23.5139) (6.1765, 23.4898) (6.166, 23.4649) (6.1538, 23.4385) (6.14, 23.4105) (6.1251, 23.381) (6.1097, 23.3507) (6.0943, 23.3201) (6.0793, 23.2897) (6.0651, 23.2593) (6.0518, 23.2289) (6.0393, 23.1981) (6.0278, 23.1665) (6.0171, 23.134) (6.0073, 23.1009) (5.9986, 23.0677) (5.991, 23.0351) (5.9845, 23.0037) (5.9794, 22.9741) (5.9754, 22.9462) (5.9724, 22.9197) (5.9703, 22.8938) (5.9689, 22.8678) (5.968, 22.841) (5.9678, 22.8128) (5.9684, 22.7832) (5.97, 22.752) (5.9729, 22.7197) (5.9771, 22.6866) (5.9824, 22.6534) (5.9887, 22.621) (5.9955, 22.59) (6.0027, 22.5613) (6.0098, 22.5353) (6.0166, 22.5127) (6.0219, 22.4972) (6.0257, 22.4872) (6.0282, 22.4813) (6.0294, 22.4784) knots 0 0 0 0 0 0 0.007407 0.014815 0.022222 0.02963 0.037037 0.044444 0.051852 0.059259 0.066667 0.074074 0.081481 0.088889 0.096296 0.103704 0.111111 0.118519 0.125926 0.133333 0.140741 0.148148 0.155556 0.162963 0.17037 0.177778 0.185185 0.192593 0.2 0.207407 0.214815 0.222222 0.22963 0.237037 0.244444 0.251852 0.259259 0.266667 0.274074 0.281481 0.288889 0.296296 0.303704 0.311111 0.318519 0.325926 0.333333 0.340741 0.348148 0.355556 0.362963 0.37037 0.377778 0.385185 0.392593 0.4 0.407407 0.414815 0.422222 0.42963 0.437037 0.444444 0.451852 0.459259 0.466667 0.474074 0.481481 0.488889 0.496296 0.503704 0.511111 0.518519 0.525926 0.533333 0.540741 0.548148 0.555556 0.562963 0.57037 0.577778 0.585185 0.592593 0.6 0.607407 0.614815 0.622222 0.62963 0.637037 0.644444 0.651852 0.659259 0.666667 0.674074 0.681481 0.688889 0.696296 0.703704 0.711111 0.718519 0.725926 0.733333 0.740741 0.748148 0.755556 0.762963 0.77037 0.777778 0.785185 0.792593 0.8 0.807407 0.814815 0.822222 0.82963 0.837037 0.844444 0.851852 0.859259 0.866667 0.874074 0.881481 0.888889 0.896296 0.903704 0.911111 0.918519 0.925926 0.933333 0.940741 0.948148 0.955556 0.962963 0.97037 0.977778 0.985185 0.992593 1 1 1 1 1 1
  spline S7 degree 5 poles (6.0294, 22.4784) (6.0315, 22.4727) (6.0358, 22.4612) (6.0425, 22.4441) (6.052, 22.4215) (6.0649, 22.3936) (6.0788, 22.3662) (6.0934, 22.3393) (6.1089, 22.3129) (6.1249, 22.2874) (6.1413, 22.2627) (6.1579, 22.2391) (6.1748, 22.2166) (6.1918, 22.1952) (6.2092, 22.1745) (6.2273, 22.1543) (6.2463, 22.1342) (6.2664, 22.1141) (6.2878, 22.0938) (6.3105, 22.0735) (6.3345, 22.0533) (6.3594, 22.0336) (6.3851, 22.0145) (6.4113, 21.9964) (6.4377, 21.9792) (6.4638, 21.9633) (6.4896, 21.9484) (6.515, 21.9347) (6.54, 21.9219) (6.5651, 21.9099) (6.5905, 21.8983) (6.6165, 21.8869) (6.6431, 21.8758) (6.6701, 21.8647) (6.6971, 21.8538) (6.7238, 21.843) (6.7499, 21.832) (6.7756, 21.8204) (6.8011, 21.8073) (6.8271, 21.7921) (6.8539, 21.774) (6.8818, 21.7526) (6.9107, 21.7281) (6.9399, 21.7012) (6.9685, 21.6728) (6.9956, 21.6439) (7.0205, 21.6157) (7.0425, 21.5887) (7.0616, 21.5631) (7.0783, 21.5385) (7.0932, 21.5143) (7.1072, 21.4896) (7.1209, 21.4638) (7.1347, 21.4366) (7.1486, 21.4078) (7.1623, 21.3778) (7.1755, 21.347) (7.1878, 21.3156) (7.199, 21.284) (7.2091, 21.2522) (7.218, 21.2201) (7.2259, 21.1878) (7.2329, 21.1551) (7.239, 21.122) (7.2444, 21.0885) (7.249, 21.0545) (7.2527, 21.0204) (7.2555, 20.986) (7.2573, 20.9517) (7.2581, 20.9173) (7.2579, 20.883) (7.2566, 20.8487) (7.2543, 20.8145) (7.251, 20.7804) (7.2467, 20.7464) (7.2415, 20.7126) (7.2355, 20.6792) (7.2287, 20.6461) (7.221, 20.6135) (7.2126, 20.5813) (7.2033, 20.5497) (7.193, 20.5184) (7.1817, 20.4876) (7.1694, 20.4571) (7.156, 20.4271) (7.1419, 20.3976) (7.1273, 20.3691) (7.1124, 20.3416) (7.0975, 20.3154) (7.0826, 20.2905) (7.0673, 20.2667) (7.0512, 20.2435) (7.0337, 20.2204) (7.0144, 20.197) (6.993, 20.1731) (6.9699, 20.1491) (6.9458, 20.1255) (6.9217, 20.1031) (6.8982, 20.0825) (6.8758, 20.0642) (6.8543, 20.0483) (6.8329, 20.0343) (6.8107, 20.0214) (6.7867, 20.0091) (6.7603, 19.9968) (6.7317, 19.9842) (6.7014, 19.9712) (6.6701, 19.9579) (6.6386, 19.9444) (6.6076, 19.9306) (6.5772, 19.9165) (6.5474, 19.9018) (6.5181, 19.8862) (6.4889, 19.8694) (6.4599, 19.8514) (6.4311, 19.8323) (6.4031, 19.8125) (6.3763, 19.7924) (6.3512, 19.7725) (6.3282, 19.7531) (6.3072, 19.7343) (6.2879, 19.7159) (6.2696, 19.6974) (6.2518, 19.6784) (6.2339, 19.6585) (6.2156, 19.637) (6.197, 19.6139) (6.1783, 19.589) (6.1597, 19.5624) (6.1416, 19.5344) (6.1244, 19.5056) (6.1083, 19.4766) (6.0937, 19.4485) (6.0807, 19.4219) (6.0695, 19.3975) (6.0601, 19.3757) (6.0543, 19.3605) (6.0507, 19.3504) (6.0488, 19.3442) (6.0479, 19.3413) knots 0 0 0 0 0 0 0.007407 0.014815 0.022222 0.02963 0.037037 0.044444 0.051852 0.059259 0.066667 0.074074 0.081481 0.088889 0.096296 0.103704 0.111111 0.118519 0.125926 0.133333 0.140741 0.148148 0.155556 0.162963 0.17037 0.177778 0.185185 0.192593 0.2 0.207407 0.214815 0.222222 0.22963 0.237037 0.244444 0.251852 0.259259 0.266667 0.274074 0.281481 0.288889 0.296296 0.303704 0.311111 0.318519 0.325926 0.333333 0.340741 0.348148 0.355556 0.362963 0.37037 0.377778 0.385185 0.392593 0.4 0.407407 0.414815 0.422222 0.42963 0.437037 0.444444 0.451852 0.459259 0.466667 0.474074 0.481481 0.488889 0.496296 0.503704 0.511111 0.518519 0.525926 0.533333 0.540741 0.548148 0.555556 0.562963 0.57037 0.577778 0.585185 0.592593 0.6 0.607407 0.614815 0.622222 0.62963 0.637037 0.644444 0.651852 0.659259 0.666667 0.674074 0.681481 0.688889 0.696296 0.703704 0.711111 0.718519 0.725926 0.733333 0.740741 0.748148 0.755556 0.762963 0.77037 0.777778 0.785185 0.792593 0.8 0.807407 0.814815 0.822222 0.82963 0.837037 0.844444 0.851852 0.859259 0.866667 0.874074 0.881481 0.888889 0.896296 0.903704 0.911111 0.918519 0.925926 0.933333 0.940741 0.948148 0.955556 0.962963 0.97037 0.977778 0.985185 0.992593 1 1 1 1 1 1
  spline S8 degree 5 poles (6.0479, 19.3413) (6.0458, 19.3355) (6.0417, 19.324) (6.0358, 19.3065) (6.0286, 19.2831) (6.0206, 19.2535) (6.0136, 19.2236) (6.0075, 19.1935) (6.0024, 19.1634) (5.9982, 19.1335) (5.9949, 19.1041) (5.9925, 19.0753) (5.991, 19.0473) (5.9902, 19.0199) (5.9903, 18.9929) (5.9911, 18.9657) (5.9928, 18.9382) (5.9953, 18.9098) (5.9986, 18.8805) (6.003, 18.8503) (6.0083, 18.8195) (6.0148, 18.7884) (6.0222, 18.7572) (6.0306, 18.7265) (6.0398, 18.6964) (6.0495, 18.6674) (6.0598, 18.6394) (6.0704, 18.6126) (6.0814, 18.5867) (6.0928, 18.5614) (6.1048, 18.5362) (6.1174, 18.5108) (6.1306, 18.4851) (6.1442, 18.4593) (6.1579, 18.4336) (6.1713, 18.4081) (6.1843, 18.3829) (6.1965, 18.3575) (6.2077, 18.3311) (6.2178, 18.3028) (6.2267, 18.2717) (6.2343, 18.2373) (6.2407, 18.2) (6.2457, 18.1606) (6.2494, 18.1205) (6.2516, 18.0809) (6.2525, 18.0433) (6.252, 18.0085) (6.2502, 17.9766) (6.2472, 17.9471) (6.2431, 17.9189) (6.238, 17.891) (6.2319, 17.8624) (6.2249, 17.8326) (6.2171, 17.8017) (6.2083, 17.7699) (6.1985, 17.7378) (6.1878, 17.7059) (6.1761, 17.6745) (6.1633, 17.6436) (6.1496, 17.6134) (6.1349, 17.5835) (6.1192, 17.554) (6.1026, 17.5247) (6.0852, 17.4955) (6.0669, 17.4666) (6.0478, 17.438) (6.0278, 17.4099) (6.0071, 17.3824) (5.9857, 17.3555) (5.9634, 17.3294) (5.9404, 17.304) (5.9166, 17.2792) (5.8922, 17.2552) (5.8671, 17.232) (5.8414, 17.2094) (5.8153, 17.1877) (5.7888, 17.1667) (5.7619, 17.1467) (5.7348, 17.1275) (5.7073, 17.1092) (5.6794, 17.0919) (5.6509, 17.0755) (5.6218, 17.0601) (5.5923, 17.0456) (5.5626, 17.0322) (5.5331, 17.0197) (5.504, 17.0082) (5.4758, 16.9977) (5.4483, 16.9883) (5.4213, 16.9798) (5.3941, 16.9724) (5.3658, 16.9659) (5.3359, 16.9604) (5.3042, 16.9559) (5.2711, 16.9524) (5.2375, 16.9498) (5.2046, 16.9481) (5.1733, 16.9474) (5.1445, 16.9478) (5.1177, 16.9494) (5.0923, 16.9524) (5.0671, 16.9569) (5.0408, 16.9629) (5.0126, 16.9704) (4.9826, 16.9791) (4.951, 16.9886) (4.9185, 16.9986) (4.8857, 17.0084) (4.8531, 17.0179) (4.8208, 17.0266) (4.7885, 17.0345) (4.7559, 17.0414) (4.7228, 17.0472) (4.689, 17.0521) (4.6547, 17.056) (4.6205, 17.0588) (4.5871, 17.0607) (4.5551, 17.0616) (4.525, 17.0615) (4.4968, 17.0606) (4.4702, 17.0589) (4.4443, 17.0565) (4.4185, 17.0534) (4.3919, 17.0496) (4.3641, 17.0449) (4.335, 17.0392) (4.3047, 17.0322) (4.2733, 17.0237) (4.2414, 17.0139) (4.2097, 17.0029) (4.1788, 16.991) (4.1495, 16.9789) (4.1224, 16.9669) (4.0982, 16.9554) (4.077, 16.9447) (4.0628, 16.9368) (4.0536, 16.9313) (4.0481, 16.9279) (4.0455, 16.9262) knots 0 0 0 0 0 0 0.007407 0.014815 0.022222 0.02963 0.037037 0.044444 0.051852 0.059259 0.066667 0.074074 0.081481 0.088889 0.096296 0.103704 0.111111 0.118519 0.125926 0.133333 0.140741 0.148148 0.155556 0.162963 0.17037 0.177778 0.185185 0.192593 0.2 0.207407 0.214815 0.222222 0.22963 0.237037 0.244444 0.251852 0.259259 0.266667 0.274074 0.281481 0.288889 0.296296 0.303704 0.311111 0.318519 0.325926 0.333333 0.340741 0.348148 0.355556 0.362963 0.37037 0.377778 0.385185 0.392593 0.4 0.407407 0.414815 0.422222 0.42963 0.437037 0.444444 0.451852 0.459259 0.466667 0.474074 0.481481 0.488889 0.496296 0.503704 0.511111 0.518519 0.525926 0.533333 0.540741 0.548148 0.555556 0.562963 0.57037 0.577778 0.585185 0.592593 0.6 0.607407 0.614815 0.622222 0.62963 0.637037 0.644444 0.651852 0.659259 0.666667 0.674074 0.681481 0.688889 0.696296 0.703704 0.711111 0.718519 0.725926 0.733333 0.740741 0.748148 0.755556 0.762963 0.77037 0.777778 0.785185 0.792593 0.8 0.807407 0.814815 0.822222 0.82963 0.837037 0.844444 0.851852 0.859259 0.866667 0.874074 0.881481 0.888889 0.896296 0.903704 0.911111 0.918519 0.925926 0.933333 0.940741 0.948148 0.955556 0.962963 0.97037 0.977778 0.985185 0.992593 1 1 1 1 1 1
  arc A7 (8.238, 22.2523) -> (7.8889, 23.3269) centre (2.2, 20.8844) ccw
  arc A8 (6.3577, 25.0136) -> (7.4118, 23.5626) centre (7.1755, 24.4993) ccw
  arc A9 (6.2808, 25.5401) -> (5.3668, 26.2042) centre (2.2, 20.8844) ccw
  arc A10 (3.1366, 26.6688) -> (4.8422, 26.1146) centre (4.1005, 26.7334) ccw
  arc A11 (2.7649, 27.0496) -> (1.6351, 27.0496) centre (2.2, 20.8844) ccw
  arc A12 (-0.4422, 26.1146) -> (1.2634, 26.6688) centre (0.2995, 26.7334) ccw
  arc A13 (-0.9668, 26.2042) -> (-1.8808, 25.5401) centre (2.2, 20.8844) ccw
  arc A14 (-3.0118, 23.5626) -> (-1.9577, 25.0136) centre (-2.7755, 24.4993) ccw
  arc A15 (-3.4889, 23.3269) -> (-3.838, 22.2523) centre (2.2, 20.8844) ccw
  arc A16 (-3.5906, 19.9877) -> (-3.5906, 21.7812) centre (-3.95, 20.8844) ccw
  arc A17 (-3.838, 19.5166) -> (-3.4889, 18.442) centre (2.2, 20.8844) ccw
  arc A18 (-1.9577, 16.7553) -> (-3.0118, 18.2062) centre (-2.7755, 17.2696) ccw
  arc A19 (-1.8808, 16.2288) -> (-0.9668, 15.5647) centre (2.2, 20.8844) ccw
  arc A20 (1.2634, 15.1001) -> (-0.4422, 15.6543) centre (0.2995, 15.0354) ccw
  arc A21 (1.6351, 14.7193) -> (2.7649, 14.7193) centre (2.2, 20.8844) ccw
  arc A22 (4.8422, 15.6543) -> (3.1366, 15.1001) centre (4.1005, 15.0354) ccw
  arc A23 (5.3668, 15.5647) -> (6.2808, 16.2288) centre (2.2, 20.8844) ccw
  arc A24 (7.4118, 18.2062) -> (6.3577, 16.7553) centre (7.1755, 17.2696) ccw
  arc A25 (7.8889, 18.442) -> (8.238, 19.5166) centre (2.2, 20.8844) ccw
  arc A26 (7.9906, 21.7812) -> (7.9906, 19.9877) centre (8.35, 20.8844) ccw
  circle A27 centre (2.2, 20.8844) radius 6.765
  arc A28 (5.3668, 26.2042) -> (4.8422, 26.1146) centre (5.1571, 25.8519) ccw
  arc A29 (6.3577, 25.0136) -> (6.2808, 25.5401) centre (6.0106, 25.2318) ccw
  arc A30 (7.8889, 23.3269) -> (7.4118, 23.5626) centre (7.5121, 23.1651) ccw
  arc A31 (7.9906, 21.7812) -> (8.238, 22.2523) centre (7.8381, 22.1617) ccw
  arc A32 (8.238, 19.5166) -> (7.9906, 19.9877) centre (7.8381, 19.6072) ccw
  arc A33 (7.4118, 18.2062) -> (7.8889, 18.442) centre (7.5121, 18.6038) ccw
  arc A34 (6.2808, 16.2288) -> (6.3577, 16.7553) centre (6.0106, 16.5371) ccw
  arc A35 (4.8422, 15.6543) -> (5.3668, 15.5647) centre (5.1571, 15.917) ccw
  arc A36 (2.7649, 14.7193) -> (3.1366, 15.1001) centre (2.7275, 15.1276) ccw
  arc A37 (1.2634, 15.1001) -> (1.6351, 14.7193) centre (1.6725, 15.1276) ccw
  arc A38 (-0.9668, 15.5647) -> (-0.4422, 15.6543) centre (-0.7571, 15.917) ccw
  arc A39 (-1.9577, 16.7553) -> (-1.8808, 16.2288) centre (-1.6106, 16.5371) ccw
  arc A40 (-3.4889, 18.442) -> (-3.0118, 18.2062) centre (-3.1121, 18.6038) ccw
  arc A41 (-3.5906, 19.9877) -> (-3.838, 19.5166) centre (-3.4381, 19.6072) ccw
  arc A42 (-3.838, 22.2523) -> (-3.5906, 21.7812) centre (-3.4381, 22.1617) ccw
  arc A43 (-3.0118, 23.5626) -> (-3.4889, 23.3269) centre (-3.1121, 23.1651) ccw
  arc A44 (-1.8808, 25.5401) -> (-1.9577, 25.0136) centre (-1.6106, 25.2318) ccw
  arc A45 (-0.4422, 26.1146) -> (-0.9668, 26.2042) centre (-0.7571, 25.8519) ccw
  arc A46 (1.6351, 27.0496) -> (1.2634, 26.6688) centre (1.6725, 26.6413) ccw
  arc A47 (3.1366, 26.6688) -> (2.7649, 27.0496) centre (2.7275, 26.6413) ccw
  circle A48 centre (2.2, 20.8844) radius 1
  point P0 (2.2, 20.8844)
  point P1 (2.2, 20.8844)
  dimension "d70" = 2
  constraints: 80 point on circle, 49 centre point, 40 tangent, 19 equal radius, 4 coincident, 2 end point, 1 horizontal, 18 other
  measures "d70" diameter of A48
extrude "Extrusion4" [suppressed]
extrude "Extrusion5" [suppressed]
equation "\"d1\" = 0.5 * d5"
equation "\"d2\" = d0"
